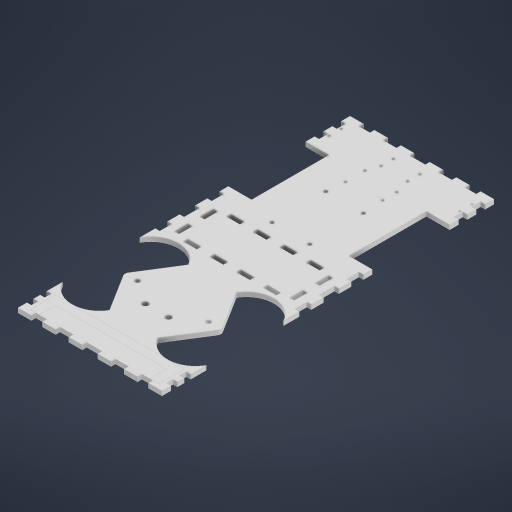
# Autodesk Inventor part: Langbektang houder
Saved by Autodesk Inventor 2023.2 (Build 272271000, 271)
## iProperties
Created: 2020-09-09
Part Number: Langbektang houder
Material: Generic
Document SubType Name: Modeling
Designer: nathan.bollaert
Density: 1 g/cm^3
Appearance: Default
Author: nathan.bollaert
Autodesk Inventor part; units mm, degrees
ref_plane "YZ Plane" through (0, 0, 0) normal (1, 0, 0) x (0, 1, 0)
ref_plane "XZ Plane" through (0, 0, 0) normal (0, 1, 0) x (-1, 0, 0)
ref_plane "XY Plane" through (0, 0, 0) normal (0, 0, 1) x (1, 0, 0)
sketch "Sketch1" plane through (0, 0, 0) normal (0, 1, 0) x (-1, 0, 0)
  line L0 (0, 0) -> (-130, 0)
  line L1 (-130, 0) -> (-130, -300)
  line L2 (-130, -300) -> (0, -300)
  line L3 (0, -40) -> (-21, -40)
  line L4 (-21, -40) -> (-21, -110)
  line L5 (-21, -110) -> (0, -110)
  line L6 (-33, -75) -> (-5.968, -56.072)
  line L7 (-5.968, -56.072) -> (-26.0432, -27.4017)
  line L8 (-26.0432, -27.4017) -> (-43.2454, -39.4468)
  line L9 (-33, -75) -> (-5.968, -93.928)
  line L10 (-5.968, -93.928) -> (-26.0432, -122.5983)
  line L11 (-43.2454, -110.5532) -> (-26.0432, -122.5983)
  arc A0 (0, -40) -> (-43.2454, -39.4468) centre (-21.7772, -51.8003) ccw
  arc A1 (-43.2454, -110.5532) -> (0, -110) centre (-21.7772, -98.1997) ccw
  line L12 (0, -75) -> (-33, -75)
  line L13 (-33, -75) -> (-21, -75)
  line L14 (-43.2454, -110.5532) -> (-22.3275, -77.1217)
  line L15 (-43.2454, -39.4468) -> (-22.3275, -72.8783)
  arc A2 (-22.3275, -77.1217) -> (-22.3275, -72.8783) centre (-25.7185, -75) ccw
  line L16 (-130, -110) -> (-109, -110)
  line L17 (-109, -110) -> (-109, -40)
  line L18 (-109, -40) -> (-130, -40)
  line L19 (-97, -75) -> (-124.032, -93.928)
  line L20 (-124.032, -93.928) -> (-103.9568, -122.5983)
  line L21 (-103.9568, -122.5983) -> (-86.7546, -110.5532)
  line L22 (-97, -75) -> (-124.032, -56.072)
  line L23 (-124.032, -56.072) -> (-103.9568, -27.4017)
  line L24 (-86.7546, -39.4468) -> (-103.9568, -27.4017)
  arc A3 (-130, -110) -> (-86.7546, -110.5532) centre (-108.2228, -98.1997) ccw
  arc A4 (-86.7546, -39.4468) -> (-130, -40) centre (-108.2228, -51.8003) ccw
  line L25 (-130, -75) -> (-97, -75)
  line L26 (-97, -75) -> (-109, -75)
  line L27 (-86.7546, -39.4468) -> (-107.6725, -72.8783)
  line L28 (-86.7546, -110.5532) -> (-107.6725, -77.1217)
  arc A5 (-107.6725, -72.8783) -> (-107.6725, -77.1217) centre (-104.2815, -75) ccw
  line L29 (0, -300) -> (0, 0)
  line L30 (0, -260) -> (-21, -260)
  line L31 (-21, -260) -> (-21, -190)
  line L32 (-21, -190) -> (0, -190)
  line L33 (0, -225) -> (-21, -225)
  line L34 (-130, -260) -> (-109, -260)
  line L35 (-109, -260) -> (-109, -190)
  line L36 (-109, -190) -> (-130, -190)
  line L37 (-109, -225) -> (-130, -225)
  point P0 (-105.3443, -69.1573)
  point P1 (-109, -66.5975)
  point P2 (-109, -83.4025)
  point P3 (-105.3443, -80.8427)
  point P4 (-24.6557, -80.8427)
  point P5 (-21, -83.4025)
  point P6 (-21, -66.5975)
  point P7 (-24.6557, -69.1573)
  point P8 (-17.2217, -40)
  point P9 (-17.2217, -110)
  point P10 (-112.7783, -40)
  point P11 (-112.7783, -110)
  dimension "d122" = 130
  dimension "d123" = 300
  dimension "d128" = 75
  dimension "d158" = 33
  dimension "d159" = 35
  dimension "d160" = 35
  dimension "d161" = 4
  dimension "d169" = 35
  dimension "d170" = 35
  dimension "d172" = 75
  dimension "d175" = 33
  dimension "d179" = 33
  dimension "d183" = 70
  dimension "d186" = 35
  dimension "d187" = 21
  dimension "d188" = 75
  dimension "d189" = 70
  dimension "d190" = 21
  dimension "d191" = 75
  dimension "d228" = 21
  constraints: 76 end point, 18 perpendicular, 17 equal length, 17 point on line, 16 point on circle, 6 centre point, 4 horizontal, 4 midpoint, 4 tangent, 3 parallel, 2 coincident, 1 equal radius, 1 vertical, 3 other
  measures "d122" distance of L2.end L1.end
  measures "d123" distance of L1.end L0.end
  measures "d128" distance of L0.start L12.start
  measures "d158" distance of L12.start L12.end
  measures "d159" angle of L12 L6
  measures "d160" angle of L9 L12
  measures "d161" radius of A2
  measures "d169" angle of L25 L19
  measures "d170" angle of L22 L25
  measures "d172" vertical distance of L0.end L25.end
  measures "d175" distance of L6.start L6.end
  measures "d179" distance from line of L23 L25.end
  measures "d183" distance between parallel lines of L18 L16
  measures "d186" distance of L20.start L20.end
  measures "d187" distance of L17.end L18.end
  measures "d188" distance of L2.end L33.start
  measures "d189" distance of L30.end L31.end
  measures "d190" distance of L30.start L30.end
  measures "d191" distance of L1.end L37.end
  measures "d228" distance of L20.end L21.end
extrude "Extrusion1" add sketch "Sketch1" along normal blind 4 contours L29 A0 L15 L6 L9 L14 A1 L32 L31 L30 L2 L1 L34 L35 L36 A3 L28 L19 L22 L27 A4 L0 | L15 A2 L12 L6 | A2 L14 L9 L12 | A5 L27 L22 L25 | L25 L19 L28 A5
sketch "Sketch2" plane through (0, 4, 0) normal (0, 1, 0) x (1, 0, 0)
  circle A0 centre (48, 181.5) radius 1.5
  circle A1 centre (48, 230) radius 1.5
  circle A2 centre (82, 230) radius 1.5
  circle A3 centre (82, 181.5) radius 1.5
  line L0 (130, 300) -> (0, 300) projected
  line L1 (0, 300) -> (0, 110) projected
  line L2 (0, 225) -> (130, 225)
  line L3 (130, 110) -> (130, 300) projected
  line L4 (0, 223.5) -> (130, 223.5)
  line L5 (130, 226.5) -> (0, 226.5)
  line L6 (0, 0) -> (130, 0) projected
  line L7 (65, 0) -> (65, 300)
  point P0 (0, 225)
  point P1 (0, 190)
  point P2 (130, 190)
  dimension "d228" = 21
  dimension "d196" = 3
  dimension "d201" = 34
  dimension "d202" = 48.5
  dimension "d205" = 75
  dimension "d208" = 3
  dimension "d209" = 5
  constraints: 6 end point, 4 centre point, 3 equal radius, 2 horizontal, 2 horizontal alignment, 2 midpoint, 2 point on line, 2 vertical alignment, 1 parallel, 1 symmetric about line, 3 other
  measures "d196" diameter of A0
  measures "d201" distance of A3.centre A0.centre
  measures "d202" distance of A0.centre A1.centre
  measures "d208" distance between parallel lines of L5 L4
hole "Hole1" at (48, 4, -181.5) at (48, 4, -230) at (82, 4, -181.5) at (82, 4, -230) direction (0, -1, 0) diameter 3 end through all
sketch "Sketch3" plane through (0, 4, 0) normal (0, 1, 0) x (1, 0, 0)
  circle A0 centre (33, 75) radius 2
  line L0 (0, 0) -> (130, 0) projected
  line L1 (0, 40) -> (0, 0) projected
  circle A1 centre (33, 75) radius 2 projected
  line L2 (65, 0) -> (65, 300)
  line L3 (130, 300) -> (0, 300) projected
  circle A2 centre (97, 75) radius 2
  dimension "d228" = 21
  dimension "d217" = 75
  dimension "d219" = 4
  dimension "d220" = 33
  constraints: 2 centre point, 2 end point, 2 midpoint, 1 other
  measures "d217" distance from line of L0 A0.centre
  measures "d219" diameter of A0
  measures "d220" distance from line of L1 A0.centre
hole "Hole2" at (33, 4, -75) at (97, 4, -75) direction (0, -1, 0) diameter 4 end through all
sketch "Sketch4" plane through (0, 4, 0) normal (0, 1, 0) x (1, 0, 0)
  circle A0 centre (54.5, 60.5) radius 2.5
  circle A1 centre (75.5, 60.5) radius 2.5
  line L0 (0, 0) -> (130, 0) projected
  line L1 (65, 0) -> (65, 300)
  line L2 (130, 300) -> (0, 300) projected
  circle A2 centre (33, 75) radius 2 projected
  dimension "d228" = 21
  dimension "d229" = 5
  dimension "d231" = 21
  dimension "d233" = 14.5
  constraints: 2 centre point, 2 end point, 2 midpoint, 1 equal radius, 1 horizontal alignment, 1 symmetric about line
  measures "d229" diameter of A0
  measures "d231" distance of A0.centre A1.centre
  measures "d233" vertical distance of A2.centre A0.centre
hole "Hole3" at (54.5, 4, -60.5) at (75.5, 4, -60.5) direction (0, -1, 0) diameter 5 end through all
sketch "Sketch5" plane through (0, 4, 0) normal (0, 1, 0) x (1, 0, 0)
  line L0 (0, 40) -> (0, 0) projected
  line L1 (0, 8) -> (4, 8)
  line L2 (4, 8) -> (4, 14)
  line L3 (4, 14) -> (0, 14)
  line L4 (0, 14) -> (0, 8)
  line L5 (0, 0) -> (130, 0) projected
  line L6 (0, 20) -> (4, 20)
  line L7 (4, 20) -> (4, 26)
  line L8 (4, 26) -> (0, 26)
  line L9 (0, 26) -> (0, 20)
  line L10 (65, 0) -> (65, 300)
  line L11 (130, 300) -> (0, 300) projected
  line L12 (0, 124) -> (4, 124)
  line L13 (4, 124) -> (4, 135)
  line L14 (4, 135) -> (0, 135)
  line L15 (0, 135) -> (0, 124)
  line L16 (0, 146) -> (4, 146)
  line L17 (4, 146) -> (4, 160)
  line L18 (4, 160) -> (0, 160)
  line L19 (0, 160) -> (0, 146)
  line L20 (0, 171) -> (4, 171)
  line L21 (4, 171) -> (4, 182)
  line L22 (0, 182) -> (0, 171)
  line L23 (4, 182) -> (0, 182)
  line L24 (21, 190) -> (0, 190) projected
  line L25 (0, 268) -> (4, 268)
  line L26 (4, 268) -> (4, 276)
  line L27 (4, 276) -> (0, 276)
  line L28 (0, 276) -> (0, 268)
  line L29 (0, 260) -> (21, 260) projected
  line L30 (0, 284) -> (4, 284)
  line L31 (4, 284) -> (4, 292)
  line L32 (4, 292) -> (0, 292)
  line L33 (0, 292) -> (0, 284)
  line L34 (130, 40) -> (130, 0)
  line L35 (130, 8) -> (126, 8)
  line L36 (126, 8) -> (126, 14)
  line L37 (126, 14) -> (130, 14)
  line L38 (130, 14) -> (130, 8)
  line L39 (130, 20) -> (126, 20)
  line L40 (126, 20) -> (126, 26)
  line L41 (126, 26) -> (130, 26)
  line L42 (130, 26) -> (130, 20)
  line L43 (130, 124) -> (126, 124)
  line L44 (126, 124) -> (126, 135)
  line L45 (126, 135) -> (130, 135)
  line L46 (130, 135) -> (130, 124)
  line L47 (130, 146) -> (126, 146)
  line L48 (126, 146) -> (126, 160)
  line L49 (130, 160) -> (130, 146)
  line L50 (126, 160) -> (130, 160)
  line L51 (130, 171) -> (126, 171)
  line L52 (126, 171) -> (126, 182)
  line L53 (130, 182) -> (130, 171)
  line L54 (126, 182) -> (130, 182)
  line L55 (109, 190) -> (130, 190)
  line L56 (130, 268) -> (126, 268)
  line L57 (126, 268) -> (126, 276)
  line L58 (126, 276) -> (130, 276)
  line L59 (130, 276) -> (130, 268)
  line L60 (130, 260) -> (109, 260)
  line L61 (130, 284) -> (126, 284)
  line L62 (126, 284) -> (126, 292)
  line L63 (130, 292) -> (130, 284)
  line L64 (126, 292) -> (130, 292)
  line L65 (12, 300) -> (22, 300)
  line L66 (22, 300) -> (22, 296)
  line L67 (22, 296) -> (12, 296)
  line L68 (12, 296) -> (12, 300)
  line L69 (34, 300) -> (46, 300)
  line L70 (46, 300) -> (46, 296)
  line L71 (46, 296) -> (34, 296)
  line L72 (34, 296) -> (34, 300)
  line L73 (58, 300) -> (72, 300)
  line L74 (72, 300) -> (72, 296)
  line L75 (72, 296) -> (58, 296)
  line L76 (58, 296) -> (58, 300)
  line L77 (84, 300) -> (96, 300)
  line L78 (96, 300) -> (96, 296)
  line L79 (96, 296) -> (84, 296)
  line L80 (84, 296) -> (84, 300)
  line L81 (108, 300) -> (118, 300)
  line L82 (118, 300) -> (118, 296)
  line L83 (118, 296) -> (108, 296)
  line L84 (108, 296) -> (108, 300)
  line L85 (12, 4) -> (22, 4)
  line L86 (22, 4) -> (22, 0)
  line L87 (22, 0) -> (12, 0)
  line L88 (12, 0) -> (12, 4)
  line L89 (46, 0) -> (34, 0)
  line L90 (46, 4) -> (46, 0)
  line L91 (34, 4) -> (46, 4)
  line L92 (34, 0) -> (34, 4)
  line L93 (72, 0) -> (58, 0)
  line L94 (72, 4) -> (72, 0)
  line L95 (58, 4) -> (72, 4)
  line L96 (58, 0) -> (58, 4)
  line L97 (96, 0) -> (84, 0)
  line L98 (96, 4) -> (96, 0)
  line L99 (84, 4) -> (96, 4)
  line L100 (84, 0) -> (84, 4)
  line L101 (118, 0) -> (108, 0)
  line L102 (118, 4) -> (118, 0)
  line L103 (108, 4) -> (118, 4)
  line L104 (108, 0) -> (108, 4)
  point P0 (0, 110)
  point P1 (130, 110)
  point P2 (0, 14)
  point P3 (130, 26)
  point P4 (58, 0)
  point P5 (72, 0)
  point P6 (84, 0)
  point P7 (96, 0)
  dimension "d228" = 21
  dimension "d242" = 6
  dimension "d244" = 4
  dimension "d245" = 6
  dimension "d246" = 6
  dimension "d252" = 11
  dimension "d253" = 14
  dimension "d256" = 14
  dimension "d257" = 11
  dimension "d259" = 11
  dimension "d263" = 11
  dimension "d264" = 8
  dimension "d265" = 8
  dimension "d266" = 8
  dimension "d267" = 8
  dimension "d268" = 8
  dimension "d269" = 8
  dimension "d272" = 12
  dimension "d273" = 10
  dimension "d274" = 12
  dimension "d275" = 14
  dimension "d276" = 12
  dimension "d277" = 10
  dimension "d278" = 12
  dimension "d279" = 12
  dimension "d280" = 12
  dimension "d281" = 12
  dimension "d282" = 12
  dimension "d284" = 10
  dimension "d285" = 12
  dimension "d286" = 14
  dimension "d287" = 12
  dimension "d288" = 10
  dimension "d294" = 12
  dimension "d295" = 12
  dimension "d296" = 12
  dimension "d297" = 12
  dimension "d298" = 12
  dimension "d299" = 12
  dimension "d300" = 14
  dimension "d301" = 8
  constraints: 200 end point, 34 parallel, 34 symmetric about line, 17 horizontal, 17 perpendicular, 16 equal length, 9 horizontal alignment, 5 vertical alignment, 4 midpoint, 3 point on line
  measures "d242" distance of L2.end L1.end
  measures "d244" distance of L1.start L1.end
  measures "d245" distance of L2.end L6.end
  measures "d246" distance of L6.end L7.end
  measures "d252" distance of L13.end L12.end
  measures "d253" vertical distance of L12.end point (0, 110)
  measures "d256" distance of L17.end L16.end
  measures "d257" distance of L16.end L13.end
  measures "d259" distance of L21.end L20.end
  measures "d263" distance of L20.end L17.end
  measures "d264" distance from line of L29 L25.end
  measures "d265" distance of L25.end L26.end
  measures "d266" distance of L30.end L31.end
  measures "d267" distance of L26.end L30.end
  measures "d268" distance from line of L11 L31.end
  measures "d269" vertical distance of L24.end L21.end
  measures "d272" distance from line of L11.end L68
  measures "d273" distance of L66.end L67.end
  measures "d274" distance of L71.start L71.end
  measures "d275" distance of L75.start L75.end
  measures "d276" distance of L79.start L79.end
  measures "d277" distance of L83.start L83.end
  measures "d278" distance of L69.start L65.end
  measures "d279" distance of L73.start L70.start
  measures "d280" distance of L77.start L74.start
  measures "d281" distance of L81.start L78.start
  measures "d282" distance of L11.start L82.start
  measures "d284" distance of L87.start L87.end
  measures "d285" distance of L89.start L92.start
  measures "d286" distance of L93.start L96.start
  measures "d287" distance of L98.end L97.end
  measures "d288" distance of L102.end L101.end
  measures "d294" distance of L0.end L87.end
  measures "d295" distance of L92.start L87.start
  measures "d296" distance of L96.start L89.start
  measures "d297" distance of L97.end L93.start
  measures "d298" distance of L101.end L98.end
  measures "d299" distance of L5.end L102.end
  measures "d300" vertical distance of L0.start L7.end
  measures "d301" distance of L0.end L1.start
extrude "Extrusion2" cut sketch "Sketch5" against normal blind 4
mark "Mark1"
sketch "Sketch7" plane through (21.7772, 4, -27.0315) normal (0, 1, 0) x (1, 0, 0)
  line L0 (-6.7772, 103.4685) -> (-6.7772, 138.4685)
  line L1 (93.2228, 138.4685) -> (93.2228, 103.4685)
  line L2 (36.2228, -23.0315) -> (50.2228, -23.0315) projected
  line L3 (43.2228, -23.0315) -> (43.2228, 268.9685)
  line L4 (50.2228, 268.9685) -> (36.2228, 268.9685) projected
  circle A0 centre (26.2228, 154.4685) radius 1.5 projected
  line L5 (-6.7772, 103.4685) -> (-10.7772, 103.4685)
  line L6 (-10.7772, 103.4685) -> (-10.7772, 115.4685)
  line L7 (-10.7772, 115.4685) -> (-6.7772, 115.4685)
  line L8 (-6.7772, 115.4685) -> (-6.7772, 103.4685)
  line L9 (-6.7772, 138.4685) -> (-10.7772, 138.4685)
  line L10 (-10.7772, 138.4685) -> (-10.7772, 126.4685)
  line L11 (-10.7772, 126.4685) -> (-6.7772, 126.4685)
  line L12 (-6.7772, 126.4685) -> (-6.7772, 138.4685)
  line L13 (1.2228, 138.4685) -> (13.2228, 138.4685)
  line L14 (13.2228, 138.4685) -> (13.2228, 142.4685)
  line L15 (13.2228, 142.4685) -> (1.2228, 142.4685)
  line L16 (1.2228, 142.4685) -> (1.2228, 138.4685)
  line L17 (25.2228, 138.4685) -> (37.2228, 138.4685)
  line L18 (37.2228, 138.4685) -> (37.2228, 142.4685)
  line L19 (37.2228, 142.4685) -> (25.2228, 142.4685)
  line L20 (25.2228, 142.4685) -> (25.2228, 138.4685)
  line L21 (49.2228, 138.4685) -> (61.2228, 138.4685)
  line L22 (61.2228, 138.4685) -> (61.2228, 142.4685)
  line L23 (61.2228, 142.4685) -> (49.2228, 142.4685)
  line L24 (49.2228, 142.4685) -> (49.2228, 138.4685)
  line L25 (-6.7772, 138.4685) -> (1.2228, 138.4685)
  line L26 (13.2228, 138.4685) -> (25.2228, 138.4685)
  line L27 (37.2228, 138.4685) -> (49.2228, 138.4685)
  line L28 (73.2228, 138.4685) -> (85.2228, 138.4685)
  line L29 (85.2228, 138.4685) -> (85.2228, 142.4685)
  line L30 (85.2228, 142.4685) -> (73.2228, 142.4685)
  line L31 (73.2228, 142.4685) -> (73.2228, 138.4685)
  line L32 (61.2228, 138.4685) -> (73.2228, 138.4685)
  line L33 (85.2228, 138.4685) -> (93.2228, 138.4685)
  line L34 (-6.7772, 120.9685) -> (93.2228, 120.9685)
  circle A1 centre (26.2228, 87.4685) radius 1.5
  line L35 (1.2228, 103.4685) -> (13.2228, 103.4685)
  line L36 (13.2228, 103.4685) -> (13.2228, 99.4685)
  line L37 (13.2228, 99.4685) -> (1.2228, 99.4685)
  line L38 (1.2228, 99.4685) -> (1.2228, 103.4685)
  line L39 (25.2228, 103.4685) -> (37.2228, 103.4685)
  line L40 (37.2228, 103.4685) -> (37.2228, 99.4685)
  line L41 (37.2228, 99.4685) -> (25.2228, 99.4685)
  line L42 (25.2228, 99.4685) -> (25.2228, 103.4685)
  line L43 (49.2228, 103.4685) -> (61.2228, 103.4685)
  line L44 (61.2228, 103.4685) -> (61.2228, 99.4685)
  line L45 (61.2228, 99.4685) -> (49.2228, 99.4685)
  line L46 (49.2228, 99.4685) -> (49.2228, 103.4685)
  line L47 (-6.7772, 103.4685) -> (1.2228, 103.4685)
  line L48 (13.2228, 103.4685) -> (25.2228, 103.4685)
  line L49 (37.2228, 103.4685) -> (49.2228, 103.4685)
  line L50 (73.2228, 99.4685) -> (73.2228, 103.4685)
  line L51 (61.2228, 103.4685) -> (73.2228, 103.4685)
  line L52 (85.2228, 103.4685) -> (85.2228, 99.4685)
  line L53 (85.2228, 99.4685) -> (73.2228, 99.4685)
  line L54 (73.2228, 103.4685) -> (85.2228, 103.4685)
  line L55 (85.2228, 103.4685) -> (93.2228, 103.4685)
  line L56 (93.2228, 103.4685) -> (93.2228, 138.4685)
  line L57 (93.2228, 103.4685) -> (97.2228, 103.4685)
  line L58 (97.2228, 103.4685) -> (97.2228, 115.4685)
  line L59 (97.2228, 115.4685) -> (93.2228, 115.4685)
  line L60 (93.2228, 115.4685) -> (93.2228, 103.4685)
  line L61 (93.2228, 138.4685) -> (97.2228, 138.4685)
  line L62 (97.2228, 138.4685) -> (97.2228, 126.4685)
  line L63 (97.2228, 126.4685) -> (93.2228, 126.4685)
  line L64 (93.2228, 126.4685) -> (93.2228, 138.4685)
  point P0 (-21.7772, -27.0315)
  point P1 (-6.7772, 115.4685)
  dimension "d228" = 21
  dimension "d313" = 35
  dimension "d316" = 12
  dimension "d318" = 12
  dimension "d319" = 100
  dimension "d320" = 4
  dimension "d321" = 12
  dimension "d323" = 8
  dimension "d324" = 12
  dimension "d326" = 16
  constraints: 126 end point, 23 symmetric about line, 13 parallel, 10 equal length, 8 horizontal, 6 perpendicular, 4 midpoint, 3 collinear, 2 point on line, 1 centre point, 2 other
  measures "d313" distance of L0.start L0.end
  measures "d316" distance of L5.end L6.end
  measures "d318" distance of L10.end L9.end
  measures "d319" distance between parallel lines of L1 L0
  measures "d320" distance between parallel lines of L6 L8
  measures "d321" distance of L15.end L14.end
  measures "d323" distance between parallel lines of L0 L16
  measures "d324" distance between parallel lines of L14 L20
  measures "d326" vertical distance of A0.centre L0.end
extrude "Extrusion3" cut sketch "Sketch7" against normal blind 4 contours L5 L6 L7 L0 | L35 L36 L37 L38 | L11 L10 L9 L0 | L39 L40 L41 L42 | L16 L15 L14 L13 | L43 L44 L45 L46 | L17 L20 L19 L18 | L24 L23 L22 L21 | L1 L61 L62 L63 | L59 L58 L57 L1 | L54 L52 L53 L50 | L31 L30 L29 L28
sketch "Sketch8" plane through (21.7772, 4, -27.0315) normal (0, 1, 0) x (1, 0, 0)
  circle A0 centre (102.2228, 247.9685) radius 1
  line L0 (87.2228, 232.9685) -> (108.2228, 232.9685) projected
  line L1 (104.2228, 256.9685) -> (104.2228, 264.9685) projected
  circle A1 centre (102.2228, 258.9685) radius 1
  line L2 (36.2228, -23.0315) -> (50.2228, -23.0315) projected
  line L3 (43.2228, -23.0315) -> (43.2228, 268.9685)
  line L4 (50.2228, 268.9685) -> (36.2228, 268.9685) projected
  circle A2 centre (-15.7772, 247.9685) radius 1
  line L5 (-0.7772, 232.9685) -> (-21.7772, 232.9685)
  line L6 (-17.7772, 256.9685) -> (-17.7772, 264.9685)
  circle A3 centre (-15.7772, 258.9685) radius 1
  circle A4 centre (55.2228, 247.9685) radius 1
  circle A5 centre (55.2228, 258.9685) radius 1
  circle A6 centre (31.2228, 258.9685) radius 1
  circle A7 centre (31.2228, 247.9685) radius 1
  point P0 (-21.7772, -27.0315)
  point P1 (97.7228, 232.9685)
  point P2 (-11.2772, 232.9685)
  dimension "d228" = 21
  dimension "d329" = 2
  dimension "d330" = 15
  dimension "d333" = 2
  dimension "d334" = 11
  dimension "d339" = 47
  constraints: 9 symmetric about line, 8 centre point, 6 end point, 3 equal radius, 3 midpoint, 2 horizontal alignment, 2 vertical alignment, 4 other
  measures "d329" diameter of A0
  measures "d330" vertical distance of point (97.723, 232.968) A0.centre
  measures "d333" distance from line of L1 A1.centre
  measures "d334" distance of A0.centre A1.centre
  measures "d339" distance of A1.centre A5.centre
hole "Hole4" at (124, 4, -275) at (124, 4, -286) at (77, 4, -275) at (77, 4, -286) at (53, 4, -275) at (53, 4, -286) at (6, 4, -275) at (6, 4, -286) direction (0, -1, 0) diameter 2 end through all
sketch "Sketch9" plane through (21.7772, 4, -27.0315) normal (0, 1, 0) x (1, 0, 0)
  circle A0 centre (27.6228, 219.3185) radius 1
  circle A1 centre (27.6228, 236.9685) radius 1
  circle A2 centre (58.8228, 221.8185) radius 1
  circle A3 centre (58.8228, 234.4685) radius 1
  line L0 (36.2228, 268.9685) -> (50.2228, 268.9685) projected
  line L1 (43.2228, 268.9685) -> (43.2228, -23.0315)
  line L2 (50.2228, -23.0315) -> (36.2228, -23.0315) projected
  line L3 (27.6228, 236.9685) -> (43.2228, 236.9685)
  line L4 (43.2228, 236.9685) -> (58.8228, 236.9685)
  point P0 (-21.7772, -27.0315)
  dimension "d228" = 21
  dimension "d341" = 2
  dimension "d342" = 17.65
  dimension "d346" = 2.5
  dimension "d347" = 2.5
  dimension "d348" = 31.2
  dimension "d349" = 32
  constraints: 6 end point, 4 centre point, 3 equal radius, 3 vertical alignment, 2 midpoint, 2 point on line, 1 collinear, 1 horizontal
  measures "d341" diameter of A1
  measures "d342" distance of A0.centre L3.start
  measures "d346" vertical distance of L3.start A3.centre
  measures "d347" vertical distance of A0.centre A2.centre
  measures "d348" distance of L3.start L4.end
  measures "d349" distance from line of L0 L3.end
hole "Hole5" at (49.4, 4, -246.35) at (49.4, 4, -264) at (80.6, 4, -261.5) at (80.6, 4, -248.85) direction (0, -1, 0) diameter 2 end through all
sketch "Sketch6" plane through (0, 4, 0) normal (0, 1, 0) x (1, 0, 0)
  line L0 (7, 4) -> (7, 27.0315)
  line L1 (7, 27.0315) -> (123, 27.0315)
  line L2 (123, 27.0315) -> (123, 4)
  line L3 (58, 296) -> (72, 296) projected
  line L4 (65, 296) -> (65, 4)
  line L5 (72, 4) -> (58, 4) projected
  arc A0 (0, 40) -> (43.2454, 39.4468) centre (21.7772, 51.8003) ccw projected
  line L6 (15, 19.0315) -> (115, 19.0315)
  line L7 (115, 19.0315) -> (115, 4)
  line L8 (15, 4) -> (15, 19.0315)
  line L9 (58, 4) -> (72, 4) projected
  line L10 (7, 4) -> (15, 4)
  line L11 (12, 4) -> (22, 4) projected
  line L12 (115, 4) -> (123, 4)
  line L13 (108, 4) -> (118, 4) projected
  point P0 (65, 4)
  point P1 (17, 4)
  point P2 (113, 4)
  point P3 (119, 4)
  dimension "d228" = 21
  dimension "d308" = 116
  dimension "d309" = 8
  dimension "d310" = 8
  dimension "d311" = 23.0315
  constraints: 19 end point, 6 midpoint, 3 horizontal, 3 perpendicular, 2 horizontal alignment, 1 coincident, 1 tangent, 1 vertical, 2 other
  measures "d308" distance between parallel lines of L2 L0
  measures "d309" distance between parallel lines of L8 L0
  measures "d310" distance between parallel lines of L1 L6
  measures "d311" distance between parallel lines of L10 L1
body "Solid4"
